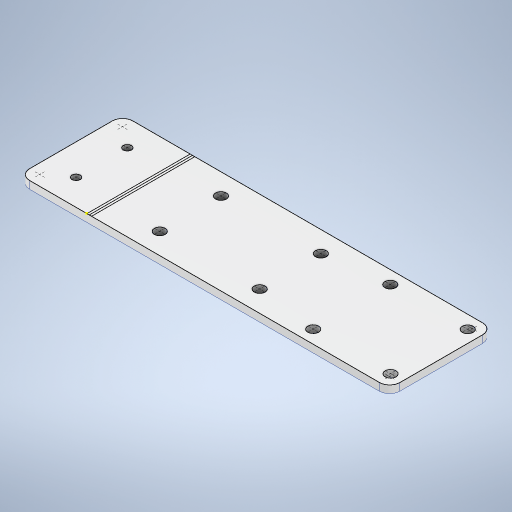
# Autodesk Inventor part: CAM_servo_bracket_bottom
Saved by Autodesk Inventor 2023 (Build 270158000, 158)
## iProperties
Created: 2022-10-29
Part Number: CAM_servo_bracket_bottom
Material: Aluminum 6061
Document SubType Name: Sheet Metal
Designer: chanh
Density: 2.7 g/cm^3
Sheet Metal Rule: Default_mm
Appearance: Aluminum - Flat
Author: chanh
Autodesk Inventor part; units mm, degrees
ref_plane "YZ Plane" through (0, 0, 0) normal (1, 0, 0) x (0, 1, 0)
ref_plane "XZ Plane" through (0, 0, 0) normal (0, 1, 0) x (-1, 0, 0)
ref_plane "XY Plane" through (0, 0, 0) normal (0, 0, 1) x (1, 0, 0)
sketch "Sketch1" plane through (0, 0, 0) normal (0, 1, 0) x (-1, 0, 0)
  line L0 (-0.4496, -20.14) -> (-0.4496, 0)
  circle A0 centre (-29.6093, -4.095) radius 1.05
  circle A1 centre (-29.6093, -16.045) radius 1.05
  circle A2 centre (-10.1093, -16.045) radius 1.05
  circle A3 centre (-10.1093, -4.095) radius 1.05
  circle A4 centre (7.19, -5.07) radius 0.7835
  circle A5 centre (7.19, -15.07) radius 0.7835
  circle A6 centre (-56.7093, -2.545) radius 1.05
  circle A7 centre (-41.6093, -2.545) radius 1.05
  circle A8 centre (-56.7093, -17.595) radius 1.05
  circle A9 centre (-41.6093, -17.595) radius 1.05
  arc A10 (-59.0893, -18.14) -> (-57.0893, -20.14) centre (-57.0893, -18.14) ccw
  line L1 (-59.0893, -2) -> (-59.0893, -18.14)
  arc A11 (-57.0893, 0) -> (-59.0893, -2) centre (-57.0893, -2) ccw
  arc A12 (11.19, -20.14) -> (13.19, -18.14) centre (11.19, -18.14) ccw
  line L2 (13.19, -2) -> (13.19, -18.14)
  arc A13 (13.19, -2) -> (11.19, 0) centre (11.19, -2) ccw
  line L3 (-57.0893, 0) -> (11.19, 0)
  line L4 (11.19, -20.14) -> (-57.0893, -20.14)
  line L5 (-0.8993, -20.14) -> (-0.8993, 0)
  line L6 (0, 0) -> (0, -20.14)
  constraints: 14 centre point, 14 end point, 11 equal radius, 8 point on circle, 8 tangent, 6 point on line, 5 vertical, 4 parallel, 2 horizontal, 2 perpendicular, 43 other
extrude "Plate1" add sketch "Sketch1" against normal blind 1.5
equation "\"d0\" = Thickness"
equation "\"BendReliefWidth\" = Thickness"
equation "\"BendReliefDepth\" = 0.5 * Thickness"
equation "\"CornerReliefSize\" = 4 * Thickness"
equation "\"MinimumRemnant\" = 2 * Thickness"
equation "\"TransitionRadius\" = BendRadius"
equation "\"JacobiRadiusSize\" = BendRadius"
equation "\"GapSize\" = Thickness"
equation "\"Thickness\" = 1.5"
equation "\"BendRadius\" = 0.31"
body "Solid1"
